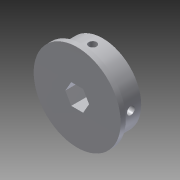
# Autodesk Inventor part: Roller End Cap Drive (3-D Printed)
Saved by Autodesk Inventor 2014 (Build 180170000, 170)
## iProperties
Created: 2014-01-12
Part Number: Roller End Cap Drive (3-D Printed)
Material: ABS Plastic
Document SubType Name: Modeling
Designer: Michael
Density: 1.06 g/cm^3
Appearance: Smooth - White
Mass: 9.04306 g
Surface Area: 41.2197 cm^2
Volume: 8.53119 cm^3
Author: Michael
Autodesk Inventor part; units mm, degrees
ref_plane "YZ Plane" through (0, 0, 0) normal (1, 0, 0) x (0, 1, 0)
ref_plane "XZ Plane" through (0, 0, 0) normal (0, 1, 0) x (-1, 0, 0)
ref_plane "XY Plane" through (0, 0, 0) normal (0, 0, 1) x (1, 0, 0)
sketch "Sketch1" plane through (0, 0, 0) normal (0, 0, 1) x (1, 0, 0)
  circle A0 centre (0, 0) radius 23.7871
  line L0 (3.6808, 6.3754) -> (7.3617, 0)
  line L1 (7.3617, 0) -> (3.6808, -6.3754)
  line L2 (3.6808, -6.3754) -> (-3.6808, -6.3754)
  line L3 (-3.6808, -6.3754) -> (-7.3617, 0)
  line L4 (-7.3617, 0) -> (-3.6808, 6.3754)
  line L5 (-3.6808, 6.3754) -> (3.6808, 6.3754)
  dimension "d0" = 47.5742
  dimension "d2" = 12.7508
  constraints: 12 end point, 2 coincident, 1 centre point, 1 horizontal, 13 other
  measures "d0" diameter of A0
  measures "d2" distance between parallel lines of L5 L2
extrude "Extrusion1" add sketch "Sketch1" along normal blind 12.7
ref_plane "Work Plane1" through (0, 23.7871, 0) normal (0, 1, 0) x (-1, 0, 0)
sketch "Sketch2" plane through (0, 23.7871, 0) normal (0, 1, 0) x (-1, 0, 0)
  line L0 (23.7871, 12.7) -> (-23.7871, 12.7) projected
  line L1 (-23.7871, 0) -> (23.7871, 0) projected
  circle A0 centre (0, 6.35) radius 2.413
  line L2 (0, 0) -> (0, 12.7) construction
  dimension "d5" = 4.826
  dimension "d6" = 6.35
  constraints: 2 end point, 2 midpoint, 1 centre point
  measures "d5" diameter of A0
  measures "d6" distance from line of A0.centre L0
extrude "Extrusion2" cut sketch "Sketch2" against normal blind 5.5563
ref_plane "Work Plane2" through (0, -23.7871, 0) normal (0, -1, 0) x (1, 0, 0)
sketch "Sketch3" plane through (0, -23.7871, 0) normal (0, -1, 0) x (1, 0, 0)
  circle A0 centre (0, 6.35) radius 2.413
  line L0 (23.7871, 12.7) -> (-23.7871, 12.7) projected
  line L1 (0, 0) -> (0, 12.7) construction
  dimension "d9" = 4.826
  dimension "d10" = 6.35
  constraints: 2 end point, 2 midpoint, 1 centre point
  measures "d9" diameter of A0
  measures "d10" distance from line of L0 A0.centre
extrude "Extrusion3" cut sketch "Sketch3" against normal blind 5.5563
ref_plane "Work Plane4" through (23.7871, 0, 0) normal (1, 0, 0) x (0, 1, 0)
ref_plane "Work Plane3" through (7.3617, 0, 0) normal (1, 0, 0) x (0, 0, 1)
sketch "Sketch4" plane through (23.7871, 0, 0) normal (1, 0, 0) x (0, 1, 0)
  line L0 (23.7871, 12.7) -> (-23.7871, 12.7) projected
  circle A0 centre (0, 6.35) radius 2.413
  line L1 (0, 0) -> (0, 12.7) construction
  dimension "d14" = 4.826
  dimension "d15" = 6.35
  constraints: 2 end point, 2 midpoint, 1 centre point
  measures "d14" diameter of A0
  measures "d15" distance from line of L0 A0.centre
extrude "Extrusion4" cut sketch "Sketch4" against normal blind 5.5563
ref_plane "Work Plane5" through (-23.7871, 0, 0) normal (1, 0, 0) x (0, 1, 0)
sketch "Sketch5" plane through (-23.7871, 0, 0) normal (1, 0, 0) x (0, 1, 0)
  line L0 (-23.7871, 0) -> (23.7871, 0) projected
  circle A0 centre (0, 6.35) radius 2.413
  line L1 (0, 12.6521) -> (0, 0) construction
  dimension "d18" = 4.826
  dimension "d19" = 6.35
  constraints: 2 end point, 1 centre point, 1 perpendicular, 1 point on line
  measures "d18" diameter of A0
  measures "d19" distance from line of L0 A0.centre
extrude "Extrusion5" cut sketch "Sketch5" along normal blind 5.5563
sketch "Sketch6" plane through (0, 0, 12.7) normal (0, 0, 1) x (1, 0, 0)
  line L0 (7.3617, 0) -> (3.6808, -6.3754) projected
  line L1 (3.6808, -6.3754) -> (-3.6808, -6.3754) projected
  line L2 (-3.6808, -6.3754) -> (-7.3617, 0) projected
  line L3 (-7.3617, 0) -> (-3.6808, 6.3754) projected
  line L4 (-3.6808, 6.3754) -> (3.6808, 6.3754) projected
  line L5 (3.6808, 6.3754) -> (7.3617, 0) projected
  circle A0 centre (0, 0) radius 23.7871 projected
  circle A1 centre (0, 0) radius 26.9621
  dimension "d26" = 3.175
  constraints: 1 centre point, 1 coincident
  measures "d26" radial gap between concentric circles of A0 A1
extrude "Extrusion6" add sketch "Sketch6" along normal blind 3.175 contours A0 | A1
fillet "Fillet1" radius 0.7937 1 edges at (-23.7871, 0, 12.7)
body "Solid1"
